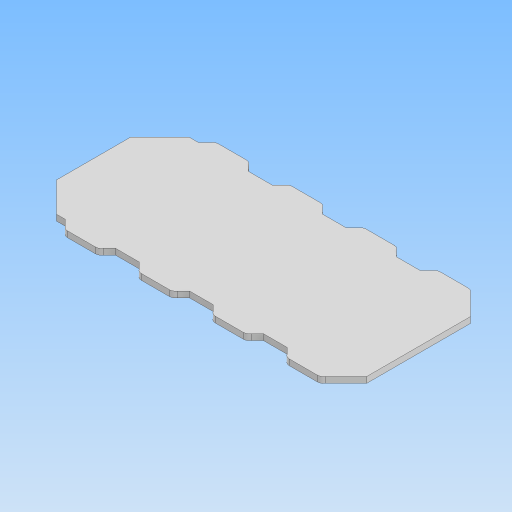
# Autodesk Inventor part: RC5 Controller kryt
Saved by Autodesk Inventor 2024 (Build 280153000, 153)
## iProperties
Created: 2024-03-14
Part Number: RC5 Controller kryt
Material: Generic
Document SubType Name: Modeling
Designer: MenMe
Density: 1 g/cm^3
Appearance: Default
Author: MenMe
Autodesk Inventor part; units mm, degrees
ref_plane "YZ Plane" through (0, 0, 0) normal (1, 0, 0) x (0, 1, 0)
ref_plane "XZ Plane" through (0, 0, 0) normal (0, 1, 0) x (-1, 0, 0)
ref_plane "XY Plane" through (0, 0, 0) normal (0, 0, 1) x (1, 0, 0)
sketch "Sketch1" plane through (0, 0, 0) normal (0, 1, 0) x (-1, 0, 0)
  arc A0 (-42.1977, 20.587) -> (-43.9298, 19.587) centre (-42.1977, 18.587) ccw
  line L0 (-45.9298, 17.587) -> (-43.9298, 19.587)
  line L1 (-50.9298, 12.587) -> (-45.9298, 17.587)
  line L2 (-50.9298, -22.413) -> (-50.9298, 12.587)
  line L3 (-43.9298, -29.413) -> (-50.9298, -22.413)
  arc A1 (-43.9298, -29.413) -> (-42.1977, -30.413) centre (-42.1977, -28.413) ccw
  line L4 (-32.6618, -30.413) -> (-42.1977, -30.413)
  arc A2 (-32.6618, -30.413) -> (-30.9298, -29.413) centre (-32.6618, -28.413) ccw
  line L5 (-28.9298, -27.413) -> (-30.9298, -29.413)
  line L6 (-20.9298, -27.413) -> (-28.9298, -27.413)
  line L7 (-18.9298, -29.413) -> (-20.9298, -27.413)
  arc A3 (-18.9298, -29.413) -> (-17.1977, -30.413) centre (-17.1977, -28.413) ccw
  line L8 (-7.6618, -30.413) -> (-17.1977, -30.413)
  arc A4 (-7.6618, -30.413) -> (-5.9298, -29.413) centre (-7.6618, -28.413) ccw
  line L9 (-3.9298, -27.413) -> (-5.9298, -29.413)
  line L10 (4.0702, -27.413) -> (-3.9298, -27.413)
  line L11 (6.0702, -29.413) -> (4.0702, -27.413)
  arc A5 (6.0702, -29.413) -> (7.8023, -30.413) centre (7.8023, -28.413) ccw
  line L12 (17.3382, -30.413) -> (7.8023, -30.413)
  arc A6 (17.3382, -30.413) -> (19.0702, -29.413) centre (17.3382, -28.413) ccw
  line L13 (21.0702, -27.413) -> (19.0702, -29.413)
  line L14 (29.0702, -27.413) -> (21.0702, -27.413)
  line L15 (31.0702, -29.413) -> (29.0702, -27.413)
  arc A7 (31.0702, -29.413) -> (32.8023, -30.413) centre (32.8023, -28.413) ccw
  line L16 (42.3382, -30.413) -> (32.8023, -30.413)
  arc A8 (42.3382, -30.413) -> (44.0702, -29.413) centre (42.3382, -28.413) ccw
  line L17 (46.0702, -27.413) -> (44.0702, -29.413)
  line L18 (49.0702, -27.413) -> (46.0702, -27.413)
  line L19 (59.0702, -17.413) -> (49.0702, -27.413)
  line L20 (59.0702, 7.587) -> (59.0702, -17.413)
  line L21 (49.0702, 17.587) -> (59.0702, 7.587)
  line L22 (46.0702, 17.587) -> (49.0702, 17.587)
  line L23 (44.0702, 19.587) -> (46.0702, 17.587)
  arc A9 (44.0702, 19.587) -> (42.3382, 20.587) centre (42.3382, 18.587) ccw
  line L24 (32.8023, 20.587) -> (42.3382, 20.587)
  arc A10 (32.8023, 20.587) -> (31.0702, 19.587) centre (32.8023, 18.587) ccw
  line L25 (29.0702, 17.587) -> (31.0702, 19.587)
  line L26 (21.0702, 17.587) -> (29.0702, 17.587)
  line L27 (19.0702, 19.587) -> (21.0702, 17.587)
  arc A11 (19.0702, 19.587) -> (17.3382, 20.587) centre (17.3382, 18.587) ccw
  line L28 (7.8023, 20.587) -> (17.3382, 20.587)
  arc A12 (7.8023, 20.587) -> (6.0702, 19.587) centre (7.8023, 18.587) ccw
  line L29 (4.0702, 17.587) -> (6.0702, 19.587)
  line L30 (-3.9298, 17.587) -> (4.0702, 17.587)
  line L31 (-5.9298, 19.587) -> (-3.9298, 17.587)
  arc A13 (-5.9298, 19.587) -> (-7.6618, 20.587) centre (-7.6618, 18.587) ccw
  line L32 (-17.1977, 20.587) -> (-7.6618, 20.587)
  arc A14 (-17.1977, 20.587) -> (-18.9298, 19.587) centre (-17.1977, 18.587) ccw
  line L33 (-20.9298, 17.587) -> (-18.9298, 19.587)
  line L34 (-28.9298, 17.587) -> (-20.9298, 17.587)
  line L35 (-30.9298, 19.587) -> (-28.9298, 17.587)
  arc A15 (-30.9298, 19.587) -> (-32.6618, 20.587) centre (-32.6618, 18.587) ccw
  line L36 (-42.1977, 20.587) -> (-32.6618, 20.587)
  point P0 (0, 0)
  point P1 (59.0702, 17.587)
  constraints: 74 end point, 32 point on circle, 16 centre point
extrude "Extrusion1" add sketch "Sketch1" along normal blind 2
body "Solid1"
